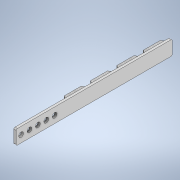
# Autodesk Inventor part: actuator_bone_joint
Saved by Autodesk Inventor 2021 (Build 250183000, 183)
## iProperties
Created: 2021-05-25
Part Number: actuator_bone_joint
Material: Generic
Document SubType Name: Modeling
Designer: Charlie
Density: 1 g/cm^3
Appearance: Default
Author: Charlie
Autodesk Inventor part; units mm, degrees
ref_plane "YZ Plane" through (0, 0, 0) normal (1, 0, 0) x (0, 1, 0)
ref_plane "XZ Plane" through (0, 0, 0) normal (0, 1, 0) x (-1, 0, 0)
ref_plane "XY Plane" through (0, 0, 0) normal (0, 0, 1) x (1, 0, 0)
sketch "Sketch3" plane through (0, 0, 0) normal (0, 1, 0) x (-1, 0, 0)
  line L0 (1, -50) -> (-1, -50)
  line L1 (-1, -50) -> (-1, 50)
  line L2 (-1, 50) -> (1, 50)
  line L3 (1, 50) -> (1, -50)
  line L4 (1, -50) -> (-1, 50) construction
  line L5 (-1, -50) -> (1, 50) construction
  line L6 (1, -50) -> (1, -30)
  line L7 (1, -30) -> (6, -30)
  line L8 (6, -30) -> (6, -50)
  line L9 (6, -50) -> (1, -50)
  line L10 (1, -30) -> (6.2137, -30) construction
  line L11 (1, -50) -> (6, -47.1132)
  line L12 (1, -50) -> (6.7735, -50) construction
  line L13 (1, -30) -> (6, -32.8868)
  line L14 (1, -30) -> (5.6279, -30) construction
  line L15 (1, -28) -> (6, -25.1132)
  line L16 (6, -8) -> (6, -28)
  line L17 (1, -8) -> (6, -10.8868)
  line L18 (1, -6) -> (6, -3.1132)
  line L19 (6, 14) -> (6, -6)
  line L20 (1, 14) -> (6, 11.1132)
  line L21 (1, 16) -> (6, 18.8868)
  line L22 (6, 36) -> (6, 16)
  line L23 (1, 36) -> (6, 33.1132)
  line L24 (-1, 50) -> (1, 50)
  line L25 (1, 50) -> (1, 80)
  line L26 (1, 80) -> (-1, 80)
  line L27 (-1, 80) -> (-1, 50)
  line L28 (-1.5102, -55) -> (-1.5102, 40) construction
  line L29 (-0.5, 40) -> (-0.6183, 40) construction
  point P0 (0, 0)
  point P1 (1, 16)
  point P2 (1, 14)
  point P3 (1, -8)
  point P4 (1, -28)
  point P5 (-1.5102, -45.1132)
  point P6 (-1.5102, -34.8868)
  point P7 (-1.5102, -12.8868)
  point P8 (-1.5102, -23.1132)
  point P9 (-1.5102, 9.1132)
  point P10 (-1.5102, -1.1132)
  point P11 (-1.5102, 31.1132)
  point P12 (-1.5102, 20.8868)
  dimension "d17" = 2
  dimension "d18" = 100
  dimension "d19" = 20
  dimension "d20" = 5
  dimension "d22" = 30
  dimension "d23" = 30
  dimension "d26" = 22
  dimension "d35" = 2
  dimension "d36" = 30
  dimension "d61" = 95
  dimension "d62" = 2
  dimension "d63" = 2
  dimension "d66" = 22
  constraints: 60 end point, 11 point on line, 6 parallel, 5 horizontal, 4 perpendicular, 2 midpoint, 2 vertical, 1 equal length, 33 other
  measures "d17" distance of L1.end L2.end
  measures "d18" distance of L0.end L1.end
  measures "d19" distance of L0.start L6.end
  measures "d20" distance of L6.end L7.end
  measures "d22" angle of L12 L11
  measures "d23" angle of L13 L14
  measures "d26" distance of L0.start L15.start
  measures "d35" distance of L26.end L25.end
  measures "d36" distance of L25.end L24.end
  measures "d61" distance of L28.start L28.end
  measures "d62" vertical distance of L11.end point (-1.51, -45.113)
  measures "d63" vertical distance of L13.end point (-1.51, -34.887)
  measures "d66" distance of point (-1.51, -34.887) point (-1.51, -12.887)
extrude "Extrusion1" add sketch "Sketch3" along normal mid plane 12 contours L0 L1 L2 L3 | L27 L26 L25 L2
extrude "Extrusion2" add sketch "Sketch3" along normal mid plane 6 contours L3 L13 L8 L11 | L3 L17 L16 L15 | L23 L22 L21 L3 | L3 L20 L19 L18
sketch "Sketch4" plane through (-1, -6, 80) normal (-1, 0, 0) x (0, 0, 1)
  circle A0 centre (-32, 6) radius 2
  line L0 (-44, 9) -> (-44, 3) projected
  line L1 (-44, 6) -> (0, 6) construction
  line L2 (0, 12) -> (0, 0) construction
  circle A1 centre (-25, 6) radius 2
  circle A2 centre (-18, 6) radius 2
  circle A3 centre (-11, 6) radius 2
  circle A4 centre (-4, 6) radius 2
  point P0 (-80, 6)
  dimension "d37" = 4
  dimension "d38" = 12
  dimension "d41" = 7
  constraints: 5 centre point, 2 end point, 2 midpoint, 1 horizontal, 8 other
  measures "d37" diameter of A0
  measures "d38" distance from line of A0.centre L0
  measures "d41" distance of A0.centre A1.centre
extrude "Extrusion3" cut sketch "Sketch4" against normal blind 6
sketch "Sketch5" plane through (-1, 6, 80) normal (0, 0, 1) x (1, 0, 0)
  line L0 (-5, -9) -> (-5, -3) construction
  line L1 (0, -9) -> (0, -3) construction
  line L2 (-5, -9) -> (0, -9) construction
  line L3 (0, -9) -> (0, -3) construction
  line L4 (0, -3) -> (-5, -3) construction
  line L5 (-5, -3) -> (-5, -9) construction
  line L6 (0, -9) -> (-5, -3) construction
  line L7 (-5, -9) -> (0, -3) construction
  line L8 (-2.5, -6) -> (-3.6, -6) construction
  line L9 (-3.6, -6) -> (-3.6, -7) construction
  circle A0 centre (-3.6, -7) radius 0.5
  circle A1 centre (-3.6, -5) radius 0.5
  point P0 (1, -6)
  dimension "d48" = 6
  dimension "d49" = 1.1
  dimension "d58" = 1
  dimension "d59" = 1
  constraints: 16 end point, 2 centre point, 2 horizontal, 2 parallel, 1 coincident, 1 midpoint, 1 perpendicular, 1 symmetric about line, 1 vertical, 1 other
  measures "d48" distance of L0.start L0.end
  measures "d49" distance of L8.start L8.end
  measures "d58" distance of L8.end L9.end
  measures "d59" diameter of A0
extrude "Extrusion4" cut sketch "Sketch5" against normal blind 150
fillet "Fillet1" radius 1 4 edges at (0, 6, 80) (0, -6, 80) (0, -6, -50) (0, 6, -50)
sketch "Sketch6" plane through (-1, -3, -50) normal (0, 0, -1) x (-1, 0, 0)
  line L0 (-2, 1) -> (-2, 5) projected
  circle A0 centre (-2, 3) radius 1
  point P0 (-1, 3)
  point P1 (-2, 4)
  point P2 (-2, 2)
  dimension "d71" = 2
  constraints: 1 centre point, 1 midpoint
  measures "d71" diameter of A0
body "Solid1"
